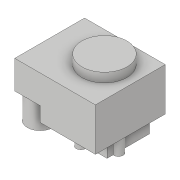
# Autodesk Inventor part: 102_Z_Focus_CCTV_Camera
Saved by Autodesk Inventor 2019 (Build 230136000, 136)
## iProperties
Created: 2019-06-18
Part Number: 102_Z_Focus_CCTV_Camera
Material: Generic
Document SubType Name: Modeling
Designer: diederichbenedict
Density: 1 g/cm^3
Appearance: Default
Author: diederichbenedict
Autodesk Inventor part; units mm, degrees
ref_plane "YZ Plane" through (0, 0, 0) normal (1, 0, 0) x (0, 1, 0)
ref_plane "XZ Plane" through (0, 0, 0) normal (0, 1, 0) x (-1, 0, 0)
ref_plane "XY Plane" through (0, 0, 0) normal (0, 0, 1) x (1, 0, 0)
sketch "Sketch1" plane through (0, 0, 0) normal (0, 1, 0) x (-1, 0, 0)
  line L0 (-15.25, 13.2) -> (15.25, 13.2)
  line L1 (15.25, 13.2) -> (15.25, -13.2)
  line L2 (15.25, -13.2) -> (-15.25, -13.2)
  line L3 (-15.25, -13.2) -> (-15.25, 13.2)
  line L4 (-15.25, 13.2) -> (15.25, -13.2) construction
  line L5 (15.25, 13.2) -> (-15.25, -13.2) construction
  point P0 (0, 0)
  dimension "d0" = 30.5
  dimension "d1" = 26.4
  constraints: 12 end point, 2 midpoint, 2 parallel, 1 horizontal, 1 perpendicular
  measures "d0" distance of L1.end L2.end
  measures "d1" distance of L0.end L1.end
extrude "Extrusion1" add sketch "Sketch1" along normal blind 16.2
sketch "Sketch2" plane through (0, 16.2, 0) normal (0, 1, 0) x (1, 0, 0)
  circle A0 centre (3.75, 1.7) radius 8.5
  line L0 (15.25, -13.2) -> (15.25, 13.2) projected
  line L1 (15.25, 13.2) -> (-15.25, 13.2) projected
  point P0 (0, 0)
  dimension "d4" = 17
  dimension "d5" = 11.5
  dimension "d6" = 11.5
  constraints: 1 centre point
  measures "d4" diameter of A0
  measures "d5" distance from line of A0.centre L0
  measures "d6" distance from line of L1 A0.centre
extrude "Extrusion2" add sketch "Sketch2" along normal blind 3.5
sketch "Sketch3" plane through (0, 0, 0) normal (0, -1, 0) x (1, 0, 0)
  line L0 (-15.25, 13.2) -> (-15.25, -13.2) projected
  line L1 (-15.25, 13.2) -> (-5.65, 13.2)
  line L2 (-5.65, 13.2) -> (-5.65, 3.6)
  line L3 (-5.65, 3.6) -> (-15.25, 3.6)
  line L4 (-15.25, 3.6) -> (-15.25, 13.2)
  point P0 (0, 0)
  dimension "d9" = 9.6
  dimension "d10" = 9.6
  constraints: 8 end point, 2 parallel, 1 horizontal, 1 perpendicular
  measures "d9" distance of L2.end L3.end
  measures "d10" distance of L1.end L2.end
extrude "Extrusion3" cut sketch "Sketch3" against normal blind 5.5
sketch "Sketch4" plane through (0, 5.5, 0) normal (0, -1, 0) x (1, 0, 0)
  line L0 (-15.25, 13.2) -> (-5.65, 13.2) projected
  line L1 (-15.25, 3.6) -> (-15.25, 13.2) projected
  line L2 (-5.65, 3.6) -> (-15.25, 3.6) projected
  line L3 (-5.65, 13.2) -> (-5.65, 3.6) projected
  circle A0 centre (-10.45, 8.4) radius 4.8
  point P0 (0, 0)
  dimension "d13" = 9.6
  constraints: 1 centre point
  measures "d13" diameter of A0
extrude "Extrusion4" add sketch "Sketch4" along normal blind 9.6 contours A0
sketch "Sketch5" plane through (0, 0, 0) normal (0, -1, 0) x (1, 0, 0)
  line L0 (-15.25, -13.2) -> (15.25, -13.2) projected
  line L1 (15.25, -13.2) -> (15.25, 13.2) projected
  line L2 (-2.25, -7.7) -> (10.75, -7.7)
  line L3 (10.75, -7.7) -> (10.75, 4.3)
  line L4 (10.75, 4.3) -> (-2.25, 4.3)
  line L5 (-2.25, 4.3) -> (-2.25, -7.7)
  arc A0 (12.75, 0.5759) -> (12.75, 4.0241) centre (13.05, 2.3) ccw
  arc A1 (2.0729, -9.7) -> (5.4271, -9.7) centre (3.75, -10.2) ccw
  arc A2 (5.2508, 6.3) -> (2.2492, 6.3) centre (3.75, 7.2) ccw
  arc A3 (-4.25, -2.7639) -> (-4.25, -5.6361) centre (-5.25, -4.2) ccw
  line L6 (12.75, -9.7) -> (5.4271, -9.7)
  line L7 (2.0729, -9.7) -> (-4.25, -9.7)
  line L8 (-15.25, 3.6) -> (-15.25, -13.2) projected
  line L9 (15.25, 13.2) -> (-5.65, 13.2) projected
  line L10 (-4.25, 6.3) -> (2.2492, 6.3)
  line L11 (5.2508, 6.3) -> (12.75, 6.3)
  line L12 (12.75, 6.3) -> (12.75, 4.0241)
  line L13 (12.75, 0.5759) -> (12.75, -9.7)
  line L14 (-4.25, -9.7) -> (-4.25, -5.6361)
  line L15 (-4.25, -2.7639) -> (-4.25, 6.3)
  point P0 (0, 0)
  dimension "d16" = 17
  dimension "d17" = 16
  dimension "d23" = 3.5
  dimension "d24" = 3.5
  dimension "d25" = 3.5
  dimension "d26" = 3.5
  dimension "d27" = 11.5
  dimension "d28" = 3
  dimension "d29" = 9
  dimension "d30" = 10
  dimension "d31" = 11.5
  dimension "d32" = 6
  dimension "d33" = 2.2
  dimension "d34" = 15.5
  constraints: 24 end point, 10 parallel, 8 point on circle, 5 perpendicular, 4 centre point, 2 horizontal
  measures "d16" distance of L10.start L11.end
  measures "d17" distance of L7.end L10.start
  measures "d23" diameter of A0
  measures "d24" diameter of A1
  measures "d25" diameter of A2
  measures "d26" diameter of A3
  measures "d27" distance from line of L1 A1.centre
  measures "d28" distance from line of A1.centre L0
  measures "d29" distance from line of A3.centre L0
  measures "d30" distance from line of A3.centre L8
  measures "d31" distance from line of A2.centre L1
  measures "d32" distance from line of A2.centre L9
  measures "d33" distance from line of A0.centre L1
  measures "d34" distance from line of L0 A0.centre
extrude "Extrusion5" add sketch "Sketch5" along normal blind 6
sketch "Sketch6" plane through (0, -6, 0) normal (0, -1, 0) x (1, 0, 0)
  line L0 (-2.25, -7.7) -> (-2.25, 4.3) projected
  line L1 (-2.25, 4.3) -> (10.75, 4.3) projected
  line L2 (10.75, 4.3) -> (10.75, -7.7) projected
  line L3 (10.75, -7.7) -> (-2.25, -7.7) projected
  line L4 (5.4271, -9.7) -> (12.75, -9.7) projected
  line L5 (12.75, -9.7) -> (12.75, 0.5759) projected
  arc A0 (12.75, 0.5759) -> (12.75, 4.0241) centre (13.05, 2.3) ccw projected
  line L6 (12.75, 4.0241) -> (12.75, 6.3) projected
  line L7 (12.75, 6.3) -> (5.2508, 6.3) projected
  arc A1 (5.2508, 6.3) -> (2.2492, 6.3) centre (3.75, 7.2) ccw projected
  line L8 (2.2492, 6.3) -> (-4.25, 6.3) projected
  line L9 (-4.25, 6.3) -> (-4.25, -2.7639) projected
  arc A2 (-4.25, -2.7639) -> (-4.25, -5.6361) centre (-5.25, -4.2) ccw projected
  line L10 (-4.25, -5.6361) -> (-4.25, -9.7) projected
  line L11 (-4.25, -9.7) -> (2.0729, -9.7) projected
  arc A3 (2.0729, -9.7) -> (5.4271, -9.7) centre (3.75, -10.2) ccw projected
  circle A4 centre (3.75, 7.2) radius 0.9
  circle A5 centre (13.05, 2.3) radius 0.9
  circle A6 centre (3.75, -10.2) radius 0.9
  circle A7 centre (-5.25, -4.2) radius 0.9
  point P0 (0, 0)
  dimension "d35" = 1.8
  dimension "d36" = 1.8
  dimension "d37" = 1.8
  constraints: 4 centre point, 4 coincident
  measures "d35" diameter of A5
  measures "d36" diameter of A6
  measures "d37" diameter of A7
extrude "Extrusion6" cut sketch "Sketch6" against normal blind 6 contours A4 | A5 | A6 | A7
body "Solid1"
